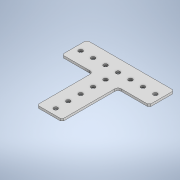
# Autodesk Inventor part: T Gusset
Saved by Autodesk Inventor 2021 (Build 250183000, 183)
## iProperties
Created: 2021-01-23
Part Number: T Gusset
Material: Generic
Document SubType Name: Modeling
Designer: aidan
Density: 1 g/cm^3
Appearance: Default
Author: aidan
Autodesk Inventor part; units mm, degrees
ref_plane "YZ Plane" through (0, 0, 0) normal (1, 0, 0) x (0, 1, 0)
ref_plane "XZ Plane" through (0, 0, 0) normal (0, 1, 0) x (-1, 0, 0)
ref_plane "XY Plane" through (0, 0, 0) normal (0, 0, 1) x (1, 0, 0)
sketch "Sketch1" plane through (0, 0, 0) normal (0, 1, 0) x (-1, 0, 0)
  line L0 (0, 0) -> (0, -57.15)
  line L1 (0, -57.15) -> (31.75, -57.15)
  line L2 (31.75, -57.15) -> (31.75, -82.55)
  line L3 (31.75, -82.55) -> (-57.15, -82.55)
  line L4 (-57.15, -82.55) -> (-57.15, -57.15)
  line L5 (-57.15, -57.15) -> (-25.4, -57.15)
  line L6 (-25.4, -57.15) -> (-25.4, 0)
  line L7 (-25.4, 0) -> (0, 0)
  dimension "d0" = 88.9
  dimension "d1" = 25.4
  dimension "d2" = 25.4
  dimension "d3" = 31.75
  dimension "d4" = 82.55
  constraints: 16 end point, 6 perpendicular, 2 point on line, 1 vertical
  measures "d0" distance between parallel lines of L4 L2
  measures "d1" distance of L1.end L2.end
  measures "d2" distance between parallel lines of L6 L0
  measures "d3" distance between parallel lines of L0 L2
  measures "d4" distance between parallel lines of L7 L3
extrude "Extrusion1" add sketch "Sketch1" along normal blind 2.286
fillet "Fillet1" radius 3.175 2 edges at (25.4, 1.143, -57.15) (0, 1.143, -57.15)
chamfer "Chamfer1" distance 1.5875 angle 45 6 edges at (0, 1.143, 0) (25.4, 1.143, 0) (57.15, 1.143, -57.15) (57.15, 1.143, -82.55) (-31.75, 1.143, -57.15) (-31.75, 1.143, -82.55)
sketch "Sketch2" plane through (0, 2.286, 0) normal (0, 1, 0) x (1, 0, 0)
  line L0 (55.5625, 82.55) -> (-30.1625, 82.55) projected
  line L1 (25.4, 1.5875) -> (25.4, 53.975) projected
  point P0 (0, 0)
  point P1 (12.7, 69.85)
  dimension "d11" = 12.7
  dimension "d12" = 12.7
  measures "d11" distance from line of L0 point (12.7, 69.85)
  measures "d12" distance from line of L1 point (12.7, 69.85)
hole "Hole1" at (12.7, 2.286, -69.85) direction (0, -1, 0) diameter 4.1402 end through all
pattern_linear "Rectangular Pattern1" count 6 spacing 12.7 along (0, 0, 1) of "Hole1"
pattern_linear "Rectangular Pattern2" count 7 spacing 12.7 along (-1, 0, 0) of "Hole1" first direction both ways yes
body "Solid1"
